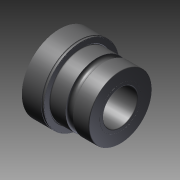
# Autodesk Inventor part: NKXZ14
Saved by Autodesk Inventor 2011 SP1 (Build 150282100, 282)
## iProperties
Created: 2016-11-23
Part Number: NKXZ14
Catalog Web Link: www.cadenas.de
Description: NKXZ-Needle Roller Bearings with Thrust Ball Bearings - With Inner Ring
Vendor: MISUMI
Document SubType Name: Modeling
Designer: psAdmin
Manufacturer: MISUMI
Mass: 10.5459 g
Surface Area: 47.5168 cm^2
Volume: 10.5459 cm^3
Density: 1 g/cm^3
Category: PARTsolutions
Company: MISUMI
Title: NKXZ14
Author: Cadenas PARTsolutions
Comments: Needle Roller Bearings with Thrust Ball Bearings - With Inner Ring
PSOL_IDENT_0: {$CADENAS_DATA\23d-libs\misumi\metric\12_bearing_holders\nkxz.prj},152 {VTYP=3D},{NB=NKXZ14},{LINA=N
PSOL_IDENT_1: KXZ14},{NN=NKXZ},{DATE=17.06.2016 05:47:22},{GEOMDATE=25.02.2016 05:06:56},{VERSION=},{LINEID=40},{L
PSOL_IDENT_2: INESUBID=-1},{WBVAR=}  {NB=NKXZ14},{LINA=NKXZ14},{KT=DUMMY},{PN=NKXZ14},{TYPE=NKXZ},{DD=14},{D=26},{
PSOL_IDENT_3: B=17},{L=25},{T=9},{RR=0.3},{RR1=0.3},{DD1=17},{D1=31.0},{LL=8.0},{AA=25.7}
NN: NKXZ
NT: Needle Roller Bearings with Thrust Ball Bearings - With Inner Ring
NB: NKXZ14
NBSYN: $PN.
LINA: NKXZ14
PN: NKXZ14
DD: 14
D: 26
B: 17
L: 25
T: 9
RR: 0.3
RR1: 0.3
DD1: 17
D1: 31.0
LL: 8.0
AA: 25.7
SUPPLIER: MISUMI
ARTICLENO: NKXZ14
BOMINFO: NKXZ14
CREATOR: CADENAS GmbH
Autodesk Inventor part; units mm, degrees
sketch "Sketch_1" plane through (0, 0, 0) normal (0, 0, 1) x (1, 0, 0)
  line L0 (25, 0) -> (0, 0)
  line L1 (0, 15.5) -> (0, 12.87)
  arc A0 (0, 12.83) -> (0, 12.87) centre (0, 12.85) ccw
  line L2 (0, 12.83) -> (0, 8.8)
  arc A1 (0, 8.8) -> (0.3, 8.5) centre (0.3, 8.8) ccw
  line L3 (0.3, 8.5) -> (8, 8.5)
  line L4 (8, 8.5) -> (8, 7)
  line L5 (8, 7) -> (24.7, 7)
  arc A2 (24.7, 7) -> (25, 7.3) centre (24.7, 7.3) ccw
  line L6 (25, 7.3) -> (25, 8.48)
  arc A3 (25, 8.52) -> (25, 8.48) centre (25, 8.5) ccw
  line L7 (25, 8.52) -> (25, 12.7)
  arc A4 (25, 12.7) -> (24.7, 13) centre (24.7, 12.7) ccw
  line L8 (24.7, 13) -> (18.5, 13)
  arc A5 (15.5, 13) -> (18.5, 13) centre (17, 13) ccw
  line L9 (15.5, 13) -> (9.3, 13)
  arc A6 (9, 13.3) -> (9.3, 13) centre (9, 13) ccw
  line L10 (9, 13.3) -> (9, 15.18)
  arc A7 (9, 15.22) -> (9, 15.18) centre (9, 15.2) ccw
  line L11 (9, 15.22) -> (9, 15.5)
  line L12 (9, 15.5) -> (8.55, 15.5)
  arc A8 (7.95, 15.5) -> (8.55, 15.5) centre (8.25, 15.5) ccw
  line L13 (7.95, 15.5) -> (0, 15.5)
  constraints: 28 end point, 18 point on circle, 9 centre point
revolve "Revolution1" add sketch "Sketch_1" angle 360 about axis through (25, 0, 0) along (1, 0, 0)
ref_plane "to_housing_XY" through (9, 0, 0) normal (1, 0, 0) x (0, 0, -1)
ref_plane "to_housing_YZ" through (9, 0, 0) normal (0, 0, -1) x (0, 1, 0)
ref_plane "to_housing_ZX" through (9, 0, 0) normal (0, 1, 0) x (1, 0, 0)
body "Solid1"
